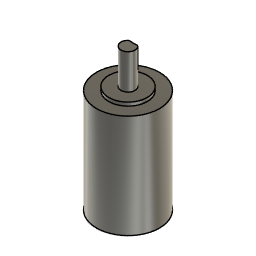
IG36P-721 (Autodesk Fusion 360 design; units mm, degrees)
Autodesk Fusion 360 part; units mm, degrees
sketch "スケッチ1" plane through (0, 0, 0) normal (0, 0, 1) x (1, 0, 0)
  circle A0 centre (0, 0) radius 18
  dimension "d1" = 36
  constraint coincident A0.centre origin
  measures "d1" diameter of A0
extrude "押し出し1" add sketch "スケッチ1" along normal blind 59.2 makes body 1
sketch "スケッチ2" plane through (0, 0, 59.2) normal (0, 0, 1) x (-1, 0, 0)
  circle A0 centre (0, 0) radius 18
  circle A1 centre (0, 0) radius 11
  dimension "d4" = 22
  constraint coincident A0.centre A1.centre
  measures "d4" diameter of A1
extrude "押し出し2" add sketch "スケッチ2" along normal blind 2 contours A1 bodies 1
sketch "スケッチ3" plane through (0, 0, 61.2) normal (0, 0, 1) x (-1, 0, 0)
  circle A0 centre (0, 0) radius 11
  circle A1 centre (0, 0) radius 4
  dimension "d7" = 8
  constraint coincident A0.centre A1.centre
  measures "d7" diameter of A1
extrude "押し出し3" add sketch "スケッチ3" along normal blind 20 contours A1 bodies 1
sketch "スケッチ4" plane through (0, 0, 81.2) normal (0, 0, 1) x (-1, 0, 0)
  circle A0 centre (0, 0) radius 4
  line L0 (0, 4) -> (0, -3)
  line L1 (0, -3) -> (-2.6458, -3)
  line L2 (0, -3) -> (0.3268, -3)
  line L3 (0.3268, -3) -> (2.6458, -3)
  dimension "d10" = 7
  constraint coincident A0 L0.start
  constraint vertical L0
  constraint coincident A0 L1.end
  constraint perpendicular L0 L1
  constraint coincident A0 L3.end
  constraint perpendicular L0 L3
  measures "d10" distance of L0.start L0.end
extrude "押し出し4" cut sketch "スケッチ4" against normal blind 12 contours A0 L1 L2 L3 bodies 1
split "分割1" by plane through (0, 0, 61.2) normal (0, 0, 1) bodies 1 makes body 2 at (3.1047, 2.5221, 67.8667)
copy_body "ボディ -> コンポーネント1" bodies 1 removing the originals makes body 3 in component "Component"
copy_body "ボディ -> コンポーネント2" bodies 2 removing the originals makes body 4 in component "Component'"
component "Component" placed x (1, 0, 0) y (0, 1, 0) z (0, 0, 1) at (0, 0, 0)
component "Component'" placed x (1, 0, 0) y (0, 1, 0) z (0, 0, 1) at (0, 0, 0)
